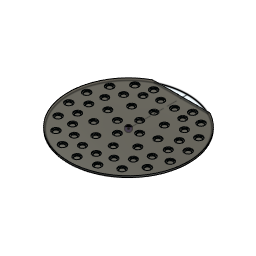
SGUv8-wormhole (Autodesk Fusion 360 design; units mm, degrees)
Autodesk Fusion 360 part; units mm, degrees
sketch "Lights" plane through (0, 0, 0) normal (0, 0, 1) x (1, 0, 0)
  circle A0 centre (0, 0) radius 80.1
  line L0 (0, 0) -> (0, 80.1) construction
  circle A1 centre (-26.0156, 59.6085) radius 5
  circle A2 centre (-26.0156, 59.6085) radius 3.5
  circle A3 centre (-44.1948, 52.6693) radius 5
  circle A4 centre (-44.1948, 52.6693) radius 3.5
  circle A5 centre (-59.5435, 34.3775) radius 5
  circle A6 centre (-59.5435, 34.3775) radius 3.5
  circle A7 centre (-67.7104, 11.9392) radius 5
  circle A8 centre (-67.7104, 11.9392) radius 3.5
  circle A9 centre (-67.7104, -11.9392) radius 5
  circle A10 centre (-67.7104, -11.9392) radius 3.5
  circle A11 centre (-59.5435, -34.3775) radius 5
  circle A12 centre (-59.5435, -34.3775) radius 3.5
  circle A13 centre (-44.1948, -52.6693) radius 5
  circle A14 centre (-44.1948, -52.6693) radius 3.5
  circle A15 centre (-23.5156, -64.6085) radius 5
  circle A16 centre (-23.5156, -64.6085) radius 3.5
  circle A17 centre (0, -68.7549) radius 5
  circle A18 centre (0, -68.7549) radius 3.5
  circle A19 centre (23.5156, -64.6085) radius 5
  circle A20 centre (23.5156, -64.6085) radius 3.5
  circle A21 centre (44.1948, -52.6693) radius 5
  circle A22 centre (44.1948, -52.6693) radius 3.5
  circle A23 centre (59.5435, -34.3775) radius 5
  circle A24 centre (59.5435, -34.3775) radius 3.5
  circle A25 centre (67.7104, -11.9392) radius 5
  circle A26 centre (67.7104, -11.9392) radius 3.5
  circle A27 centre (67.7104, 11.9392) radius 5
  circle A28 centre (67.7104, 11.9392) radius 3.5
  circle A29 centre (59.5435, 34.3775) radius 5
  circle A30 centre (59.5435, 34.3775) radius 3.5
  circle A31 centre (44.1948, 52.6693) radius 5
  circle A32 centre (44.1948, 52.6693) radius 3.5
  circle A33 centre (26.0156, 59.6085) radius 5
  circle A34 centre (26.0156, 59.6085) radius 3.5
  line L1 (0, 0) -> (-80.1, 0) construction
  circle A35 centre (-44.1948, 52.6693) radius 5
  circle A36 centre (-44.1948, 52.6693) radius 3.5
  circle A37 centre (-53, 0) radius 4.7797
  circle A38 centre (-53, 0) radius 3.2906
  circle A39 centre (-53, 0) radius 4.7797
  circle A40 centre (-53, 0) radius 3.2906
  circle A41 centre (-53, 0) radius 4.7797
  circle A42 centre (-53, 0) radius 3.2906
  circle A43 centre (-53, 0) radius 4.7797
  circle A44 centre (-53, 0) radius 3.2906
  circle A45 centre (-53, 0) radius 4.7797
  circle A46 centre (-53, 0) radius 3.2906
  circle A47 centre (-53, 0) radius 4.7797
  circle A48 centre (-53, 0) radius 3.2906
  circle A49 centre (-53, 0) radius 4.7797
  circle A50 centre (-53, 0) radius 3.2906
  circle A51 centre (-53, 0) radius 4.7797
  circle A52 centre (-53, 0) radius 3.2906
  circle A53 centre (-53, 0) radius 4.7797
  circle A54 centre (-53, 0) radius 3.2906
  circle A55 centre (-49.8037, -18.1271) radius 4.7797
  circle A56 centre (-49.8037, -18.1271) radius 3.2906
  circle A57 centre (-40.6004, -34.0677) radius 4.7797
  circle A58 centre (-40.6004, -34.0677) radius 3.2906
  circle A59 centre (-26.5, -45.8993) radius 4.7797
  circle A60 centre (-26.5, -45.8993) radius 3.2906
  circle A61 centre (-9.2034, -52.1948) radius 4.7797
  circle A62 centre (-9.2034, -52.1948) radius 3.2906
  circle A63 centre (9.2034, -52.1948) radius 4.7797
  circle A64 centre (9.2034, -52.1948) radius 3.2906
  circle A65 centre (26.5, -45.8993) radius 4.7797
  circle A66 centre (26.5, -45.8993) radius 3.2906
  circle A67 centre (40.6004, -34.0677) radius 4.7797
  circle A68 centre (40.6004, -34.0677) radius 3.2906
  circle A69 centre (49.8037, -18.1271) radius 4.7797
  circle A70 centre (49.8037, -18.1271) radius 3.2906
  circle A71 centre (53, 0) radius 4.7797
  circle A72 centre (53, 0) radius 3.2906
  circle A73 centre (49.8037, 18.1271) radius 4.7797
  circle A74 centre (49.8037, 18.1271) radius 3.2906
  circle A75 centre (40.6004, 34.0677) radius 4.7797
  circle A76 centre (40.6004, 34.0677) radius 3.2906
  circle A77 centre (26.5, 45.8993) radius 4.7797
  circle A78 centre (26.5, 45.8993) radius 3.2906
  circle A79 centre (9.2034, 52.1948) radius 4.7797
  circle A80 centre (9.2034, 52.1948) radius 3.2906
  circle A81 centre (-9.2034, 52.1948) radius 4.7797
  circle A82 centre (-9.2034, 52.1948) radius 3.2906
  circle A83 centre (-26.5, 45.8993) radius 4.7797
  circle A84 centre (-26.5, 45.8993) radius 3.2906
  circle A85 centre (-40.6004, 34.0677) radius 4.7797
  circle A86 centre (-40.6004, 34.0677) radius 3.2906
  circle A87 centre (-49.8037, 18.1271) radius 4.7797
  circle A88 centre (-49.8037, 18.1271) radius 3.2906
  circle A89 centre (0, 34) radius 4.7801
  circle A90 centre (0, 34) radius 3.2911
  circle A91 centre (-21.8548, 26.0455) radius 4.7801
  circle A92 centre (-21.8548, 26.0455) radius 3.2911
  circle A93 centre (-33.4835, 5.904) radius 4.7801
  circle A94 centre (-33.4835, 5.904) radius 3.2911
  circle A95 centre (-29.4449, -17) radius 4.7801
  circle A96 centre (-29.4449, -17) radius 3.2911
  circle A97 centre (-11.6287, -31.9495) radius 4.7801
  circle A98 centre (-11.6287, -31.9495) radius 3.2911
  circle A99 centre (11.6287, -31.9495) radius 4.7801
  circle A100 centre (11.6287, -31.9495) radius 3.2911
  circle A101 centre (29.4449, -17) radius 4.7801
  circle A102 centre (29.4449, -17) radius 3.2911
  circle A103 centre (33.4835, 5.904) radius 4.7801
  circle A104 centre (33.4835, 5.904) radius 3.2911
  circle A105 centre (21.8548, 26.0455) radius 4.7801
  circle A106 centre (21.8548, 26.0455) radius 3.2911
  circle A107 centre (0, 14.8675) radius 4.7801
  circle A108 centre (0, 14.8675) radius 3.2911
  circle A109 centre (-14.8675, 0) radius 4.7801
  circle A110 centre (-14.8675, 0) radius 3.2911
  circle A111 centre (0, -14.8675) radius 4.7801
  circle A112 centre (0, -14.8675) radius 3.2911
  circle A113 centre (14.8675, 0) radius 4.7801
  circle A114 centre (14.8675, 0) radius 3.2911
  line L2 (38.3, 70.35) -> (-38.3, 70.35)
  line L3 (0, 70.35) -> (0, -80.1) construction
  point P0 (38.3, 70.35)
  point P1 (-38.3, 70.35)
  dimension "d1" = 160.2
  dimension "d9" = 360
  dimension "d10" = 53
  dimension "d12" = 360
  dimension "d14" = 360
  dimension "d15" = 34
  dimension "d19" = 360
  dimension "d30" = 9.75
  constraint coincident A0.centre L0.start
  constraint coincident A0 L0.end
  constraint vertical L0
  constraint coincident A0 L1.end
  constraint perpendicular L0 L1
  constraint coincident L1 A37.centre
  constraint coincident A37.centre A38.centre
  constraint coincident A89.centre A90.centre
  constraint coincident L0 A89.centre
  constraint coincident A107.centre A108.centre
  constraint coincident A0 P0
  constraint coincident A0 P1
  constraint horizontal L2
  constraint midpoint L2 L3.start
  constraint coincident A0 L3.end
  constraint perpendicular L2 L3
  constraint coincident P0 L2.start
  constraint coincident P1 L2.end
  measures "d1" diameter of A0
  measures "d10" distance of A0.centre A37.centre
  measures "d15" distance of A0.centre A89.centre
  measures "d30" distance of L0.end L2
extrude "Extrude1" add sketch "Lights" along normal blind 2 contours A0 L2 picked at (12.9184, 13.8467) makes body 1
extrude "Extrude2" add sketch "Lights" along normal blind 0.75 contours A1 | A3 A35 | A5 | A7 | A9 | A11 | A13 | A15 | A17 | A19 | A21 | A23 | A25 | A27 | A29 | A31 | A33 | A34 | A37 A39 A41 A43 A45 A47 A49 A51 A53 | A55 | A57 | A59 | A61 | A63 | A65 | A67 | A69 | A71 | A73 | A75 | A77 | A79 | A81 | A83 | A85 | A87 | A89 | A91 | A93 | A95 | A97 | A99 | A101 | A103 | A105 | A107 | A109 | A111 | A113 bodies 1
extrude "Extrude11" cut sketch "Lights" along normal up to surface (0.75 mm away) contours A34 bodies 1
sketch "Sketch1" plane through (0, 0, 0) normal (0, 0, 1) x (1, 0, 0) in component "Outer-rim"
  line L0 (40.1482, 70.35) -> (-40.1482, 70.35)
  line L1 (38.3, 70.35) -> (-38.3, 70.35)
  arc A0 (-40.1482, 70.35) -> (40.1482, 70.35) centre (0, 0) ccw
  arc A1 (-41.5726, 68.35) -> (41.5726, 68.35) centre (0, 0) ccw
  line L2 (2, 68.35) -> (2, 70.3502)
  line L3 (-2, 68.35) -> (-2, 70.35)
  line L4 (0, 70.35) -> (0, -80.1)
  line L5 (2, 68.35) -> (43.4658, 68.35)
  line L6 (-2, 68.35) -> (-43.4658, 68.35)
  arc A2 (-35.4581, 68.35) -> (35.4581, 68.35) centre (0, 0) ccw
  dimension "d90" = 162
  dimension "d91" = 160
  dimension "d92" = 70.35
  dimension "d95" = 2
  dimension "d96" = 2
  dimension "d100" = 154
  dimension "d101" = 2
  dimension "d102" = 2
  constraint coincident A0.centre A1.centre
  constraint horizontal L0
  constraint vertical L2
  constraint coincident L1 L3.end
  constraint perpendicular L1 L3
  constraint concentric A0 A2
  constraint coincident A0 L5.end
  constraint perpendicular L2 L5
  constraint coincident A0 L6.end
  constraint perpendicular L3 L6
  constraint coincident L5 A1.end
  constraint coincident L5 A2.end
  constraint coincident L6 A2.start
  constraint coincident L6 A1.start
  measures "d90" diameter of A0
  measures "d91" diameter of A1
  measures "d92" distance of A0.centre L0
  measures "d95" distance of L3 L4
  measures "d96" distance of L2 L4
  measures "d100" diameter of A2
  measures "d101" distance of L0 L5
  measures "d102" distance of L0 L6
extrude "Extrude1'" add sketch "Sketch1" against normal blind 2 separate body contours L0 L1 A0 L2 L5 | A0 A1 L5 L6 | L0 L1 A0 L3 L6 | A1 L4 L5 A2 | A1 L4 L6 A2 makes body 2 in component "Outer-rim"
extrude "Extrude2'" add sketch "Sketch1" against normal blind 8 contours L0 L1 A0 L2 L5 | A0 A1 L5 L6 | L0 L1 A0 L3 L6 bodies 2 in component "Outer-rim"
chamfer "Chamfer1" distance 2 angle 45 2 edges at (2, 68.35, -4) (-2, 68.35, -4) on bodies 2 in component "Outer-rim"
sketch "Sketch2" plane through (0, 0, 0) normal (0, 0, 1) x (1, 0, 0) in component "filter"
  circle A0 centre (0, 0) radius 78.75
  line L0 (35.5879, 70.25) -> (-35.5879, 70.25)
  line L1 (0, 0) -> (0, 78.75) construction
  dimension "d108" = 157.5
  dimension "d111" = 8.5
  dimension "d111" = 8.5
  constraint coincident A0.centre L1.start
  constraint coincident A0 L0.start
  constraint coincident A0 L0.end
  constraint horizontal L0
  constraint coincident A0 L1.end
  constraint perpendicular L0 L1
  measures "d108" diameter of A0
  measures "d111" distance of L0 L1.end
extrude "Extrude2''" add sketch "Sketch2" along normal blind 0.5 separate body contours A0 L0 picked at (3.3048, 19.4447) makes body 3 in component "filter"
component "filter" placed x (1, 0, 0) y (0, 1, 0) z (0, 0, 1) at (0, 0, 0)
component "Outer-rim" placed x (1, 0, 0) y (0, 1, 0) z (0, 0, 1) at (0, 0, 0)
equation "d1 = 80.1 * 2 mm"
equation "d90 = ( 81 * 2 ) * 1 mm"
equation "d108 = ( 78.75 * 2 ) * 1 mm"
named bodies: "Wormhole", "Outer-rim", "Filter"
